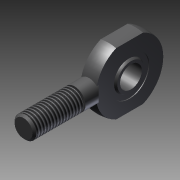
# Autodesk Inventor part: SA 12 E
Saved by Autodesk Inventor 2016 SP1 (Build 200210100, 210)
## iProperties
Category: PARTsolutions
Company: SKF
Created: 2016-06-12
Part Number: SA 12 E
Catalog Web Link: www.cadenas.de
Description: AHR_003-Rod ends with a male thread
Vendor: SKF
Document SubType Name: Modeling
Designer: psAdmin
Manufacturer: SKF
Mass: 78 g
Surface Area: 47.79 cm^2
Volume: 12.2167 cm^3
Density: 1 g/cm^3
Material: Generic
Appearance: PSOLRGB-175-175-175
PSOL_IDENT_0: {$CADENAS_DATA\23d-libs\skf\bearings_units_and_housings\plain_bearings\rod_ends\ahr_003.prj},160 {VT
PSOL_IDENT_1: YP=3D},{NB=SA 12 E},{LINA=SA 12 E},{NN=AHR_003},{DATE=19.05.2016 08:16:52},{GEOMDATE=13.05.2016 10:2
PSOL_IDENT_2: 3:42},{VERSION=},{LINEID=18090},{LINESUBID=-1},{WBVAR=}  {NB=SA 12 E},{LINA=SA 12 E},{KT=DUMMY},{PRO
PSOL_IDENT_3: DUCTID=208020006},{DESIGNATION=SA 12 E},{DD=12.000},{B=10.000},{DDK=18.000},{G=M 12},{C1=8.500},{DD2=
PSOL_IDENT_4: 35.000},{HH=54.000},{LL1=28.000},{LL2=73.000},{LL7=17.000},{R1=0.300},{AT=10.000},{LOAD1=10.800},{LO
PSOL_IDENT_5: AD2=24.500},{MASS=0.078},{TYPEID=208020},{TAXONOMY=1},{BZ=12},{GALG=0.5},{TP=1.75},{DESIGN=rodend_ma
PSOL_IDENT_6: le1},{MAPPING=BAZ50,DESIGNATION|IRD01,DD|IRL01,B|IRD20,DDK|HOT01,G|HOL01A,C1|HOD01A,DD2|HOL35,HH|HOL
PSOL_IDENT_7: 50B,LL1|HOL40A,LL2|HOL10B,LL7|IRR20,R1|BCA10,AT|BCC02,LOAD1|HOC16,LOAD2|BAM01,MASS},{DESIGNLIST=rode
PSOL_IDENT_8: nd_male1,rodend_male1x},{SORT=DD},{PIM=SA 12 E}
NN: AHR_003
NT: Rod ends with a male thread
NB: SA 12 E
NBSYN: $DESIGNATION.
LINA: SA 12 E
DESIGNATION: SA 12 E
DD: 12.000
B: 10.000
G: M 12
C1: 8.500
DD2: 35.000
HH: 54.000
AT: 10.000
LOAD1: 10.800
LOAD2: 24.500
SUPPLIER: SKF
ARTICLENO: SA 12 E
BOMINFO: SA 12 E
CREATOR: CADENAS GmbH
Title: SA 12 E
Author: Cadenas PARTsolutions
Comments: Rod ends with a male thread
Autodesk Inventor part; units mm, degrees
ref_plane "YZ Plane" through (0, 0, 0) normal (1, 0, 0) x (0, 1, 0)
ref_plane "XZ Plane" through (0, 0, 0) normal (0, 1, 0) x (-1, 0, 0)
ref_plane "XY Plane" through (0, 0, 0) normal (0, 0, 1) x (1, 0, 0)
sketch "Sketch_1" plane through (0, 0, 0) normal (0, 0, 1) x (1, 0, 0)
  line L0 (100, 0) -> (-100, 0)
  line L1 (0, 6) -> (10, 6)
  line L2 (10, 6) -> (10, 7.4833)
  arc A0 (10, 7.4833) -> (8.825, 8.1467) centre (5, 0) ccw
  line L3 (8.825, 8.1467) -> (8.825, 10.8)
  line L4 (8.825, 10.8) -> (9.25, 10.8)
  line L5 (9.25, 10.8) -> (9.25, 18.5186)
  arc A1 (9.25, 18.5186) -> (0.75, 18.5186) centre (5, 0) ccw
  line L6 (0.75, 18.5186) -> (0.75, 10.8)
  line L7 (0.75, 10.8) -> (1.175, 10.8)
  line L8 (1.175, 10.8) -> (1.175, 8.1467)
  arc A2 (1.175, 8.1467) -> (0, 7.4833) centre (5, 0) ccw
  line L9 (0, 7.4833) -> (0, 6)
  constraints: 20 end point, 6 point on circle, 3 centre point
revolve "Revolution1" add sketch "Sketch_1" angle 360 about axis through (100, 0, 0) along (1, 0, 0)
sketch "Sketch_4" plane through (0, 0, 0) normal (0, 1, 0) x (-1, 0, 0)
  line L0 (30, 35) -> (-40, 35)
  line L1 (-40, 35) -> (-40, -35)
  line L2 (-40, -35) -> (30, -35)
  line L3 (30, -35) -> (30, 35)
  circle A0 centre (-5, 0) radius 17.5
  constraints: 8 end point, 1 centre point
extrude "Extrusion1" cut sketch "Sketch_4" along normal mid plane 70
sketch "Sketch_2" plane through (0, 0, 0) normal (0, 0, 1) x (1, 0, 0)
  line L0 (5, -26) -> (5, -11.7)
  line L1 (5, -11.7) -> (11, -11.7)
  line L2 (11, -11.7) -> (11, -26)
  line L3 (11, -26) -> (5, -26)
  line L4 (5, -26) -> (5, -11.7)
  constraints: 10 end point
revolve "Revolution2" add sketch "Sketch_2" angle 360 about axis through (5, -26, 0) along (0, -1, 0)
sketch "Sketch_6" plane through (0, 0, 0) normal (0, 0, 1) x (1, 0, 0)
  line L0 (5, -54) -> (5, -26)
  line L1 (5, -26) -> (9.9265, -26)
  line L2 (9.9265, -26) -> (11, -27.0735)
  line L3 (11, -27.0735) -> (11, -52.9265)
  line L4 (11, -52.9265) -> (9.9265, -54)
  line L5 (9.9265, -54) -> (5, -54)
  line L6 (5, -54) -> (5, -26)
  constraints: 14 end point
revolve "Revolution3" add sketch "Sketch_6" angle 360 about axis through (5, -54, 0) along (0, -1, 0)
thread "Thread1" size "M12x1.75" class "6g" standard "ISO Metric profile" full length
sketch "Sketch_3" plane through (0, 0, 0) normal (0, 0, 1) x (1, 0, 0)
  line L0 (9.25, -17) -> (21.25, -29)
  line L1 (21.25, -29) -> (21.25, -11.7)
  line L2 (21.25, -11.7) -> (9.25, -11.7)
  line L3 (9.25, -11.7) -> (9.25, -17)
  constraints: 8 end point
extrude "Extrusion2" cut sketch "Sketch_3" along normal mid plane 70
sketch "Sketch_5" plane through (0, 0, 0) normal (0, 0, 1) x (1, 0, 0)
  line L0 (-11.25, -29) -> (0.75, -17)
  line L1 (0.75, -17) -> (0.75, -11.7)
  line L2 (0.75, -11.7) -> (-11.25, -11.7)
  line L3 (-11.25, -11.7) -> (-11.25, -29)
  constraints: 8 end point
extrude "Extrusion3" cut sketch "Sketch_5" along normal mid plane 70
body "Solid1"
